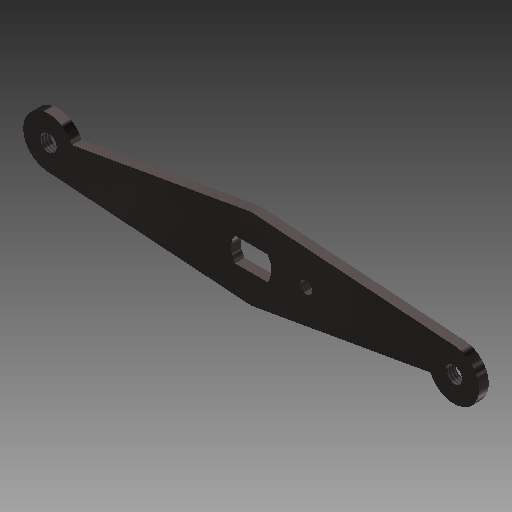
# Autodesk Inventor part: 406-01
Saved by Autodesk Inventor 2019 (Build 230136000, 136)
## iProperties
Company: Autodesk Inc.
Created: 2017-06-27
Part Number: 406-01
Material: Aluminum-6061
Document SubType Name: Modeling
Designer: Autodesk Inc.
Mass: 4.77902 g
Surface Area: 23.3131 cm^2
Volume: 1.77001 cm^3
Density: 2.7 g/cm^3
Appearance: Anodized - Subtle Dark Bronze
Author: Inventor
Autodesk Inventor part; units mm, degrees
ref_plane "YZ Plane" through (0, 0, 0) normal (1, 0, 0) x (0, 1, 0)
ref_plane "XZ Plane" through (0, 0, 0) normal (0, 1, 0) x (-1, 0, 0)
ref_plane "XY Plane" through (0, 0, 0) normal (0, 0, 1) x (1, 0, 0)
sketch "Sketch1" plane through (0, 0, 0) normal (0, 0, 1) x (1, 0, 0)
  line L0 (0, 8) -> (0, -8)
  line L1 (0, 8) -> (40.3488, 5.1785)
  arc A0 (35.3957, -1.7588) -> (40.3488, 5.1785) centre (40, 0.1907) ccw
  line L2 (35.3957, -1.7588) -> (0, -8)
  line L3 (0, 0) -> (-17.0336, 0) construction
  dimension "d0" = 16
  dimension "d1" = 10
  dimension "d2" = 14
  dimension "d3" = 40
  dimension "d4" = 10
  dimension "d5" = 7.8093
  constraints: 8 end point, 2 point on circle, 1 centre point, 1 coincident, 1 midpoint, 1 perpendicular, 1 tangent, 1 vertical
  measures "d0" distance of L0.start L0.end
  measures "d1" angle of L3 L2
  measures "d2" angle of L1 L2
  measures "d3" distance from line of L0 A0.centre
  measures "d4" diameter of A0
  measures "d5" vertical distance of L0.start A0.centre
extrude "Extrusion1" add sketch "Sketch1" along normal blind 1.9
hole "Hole1" at (40, 0.1907, 1.9) direction (0, 0, -1) diameter 3.25 end through all
thread "Thread1" size "M3.5x0.6" class "6H" standard "ANSI Metric M Profile" full length
pattern_circular "Circular Pattern1" count 2 over 360 about axis through (0, 0, -10) along (0, 0, 1)
sketch "Sketch2" plane through (0, 0, 1.9) normal (0, 0, 1) x (1, 0, 0)
  circle A0 centre (0, 0) radius 4
  line L0 (-3.2186, 2.375) -> (3.2186, 2.375)
  line L1 (3.2186, -2.375) -> (-3.2186, -2.375)
  dimension "d20" = 8
  dimension "d21" = 4.75
  constraints: 4 end point, 4 point on circle, 2 parallel, 1 centre point, 1 coincident, 1 horizontal
  measures "d20" diameter of A0
  measures "d21" distance between parallel lines of L0 L1
extrude "Extrusion2" cut sketch "Sketch2" against normal through all contours A0 L1 L0
sketch "Sketch3" plane through (0, 0, 1.9) normal (0, 0, 1) x (1, 0, 0)
  point P0 (0, 0)
  point P1 (10.843, 0.5)
  dimension "d24" = 10.843
  dimension "d25" = 0.5
  measures "d24" horizontal distance of point (0, 0) point (10.843, 0.5)
  measures "d25" vertical distance of point (10.843, 0.5) point (0, 0)
hole "Hole2" at (10.843, 0.5, 1.9) direction (0, 0, -1) diameter 2.459 end through all thread size "M3x0.5" class "6H" standard "ANSI Metric M Profile"
body "Solid1"
